Sholder Mount_v3 (Autodesk Fusion 360 design; units mm, degrees)
Autodesk Fusion 360 part; units mm, degrees
sketch "Sketch1" plane through (0, 0, 0) normal (0, 0, 1) x (1, 0, 0)
  circle A0 centre (0, 0) radius 65.25
  circle A1 centre (0, 0) radius 74.419 construction
  circle A2 centre (0, 74.419) radius 1.5
  circle A3 centre (-64.4487, -37.2095) radius 1.5
  circle A4 centre (64.4487, -37.2095) radius 1.5
  circle A5 centre (0, 0) radius 80
  line L0 (-80, 0) -> (80, 0) construction
  line L1 (-80, 0) -> (-80, -85)
  line L2 (80, -85) -> (80, 0)
  line L3 (-80, -95) -> (-100, -95) construction
  line L4 (-100, -95) -> (-90, -95)
  line L5 (100, -95) -> (100, -105)
  line L6 (100, -105) -> (-100, -105)
  line L7 (-100, -105) -> (-100, -95)
  arc A6 (-90, -95) -> (-80, -85) centre (-90, -85) ccw
  line L8 (90, -95) -> (100, -95)
  arc A7 (80, -85) -> (90, -95) centre (90, -85) ccw
  line L9 (-100, -100) -> (-30, -100) construction
  line L10 (-100, -100) -> (40, -100) construction
  circle A8 centre (-30, -100) radius 1.5
  circle A9 centre (40, -100) radius 1.5
  dimension "d1" = 130.5
  dimension "d4" = 148.838
  dimension "d5" = 3
  dimension "d7" = 360
  dimension "d8" = 160
  dimension "d10" = 200
  dimension "d11" = 10
  dimension "d12" = 10
  dimension "d13" = 10
  dimension "d22" = 105
  dimension "d24" = 70
  dimension "d25" = 140
  dimension "d26" = 3
  dimension "d27" = 3
  constraint coincident A0.centre A1.centre
  constraint concentric A0 A1
  constraint coincident A1 A2.centre
  constraint concentric A1 A5
  constraint coincident A5 L0.start
  constraint coincident A5 L0.end
  constraint horizontal L0
  constraint tangent A5 L1
  constraint perpendicular L0 L1
  constraint tangent A5 L2
  constraint perpendicular L1 L3
  constraint horizontal L4
  constraint vertical L5
  constraint horizontal L6
  constraint vertical L7
  constraint coincident L3.start L1
  constraint coincident L5.start L4
  constraint tangent L1 A6
  constraint tangent L4 A6
  constraint perpendicular L5 L8
  constraint tangent L8 A7
  constraint tangent L2 A7
  constraint midpoint L7 L9.start
  constraint perpendicular L7 L9
  constraint perpendicular L7 L10
  constraint coincident L9.end A8.centre
  constraint coincident L10.end A9.centre
  measures "d1" diameter of A0
  measures "d4" diameter of A1
  measures "d5" diameter of A2
  measures "d8" diameter of A5
  measures "d10" distance of L3.end L5.start
  measures "d11" distance of L3.end L6.end
  measures "d12" radius of A6 L3.start
  measures "d13" radius of A7
  measures "d22" distance of A0.centre L6
  measures "d24" distance of L9.start L9.end
  measures "d25" distance of L9.start L10.end
  measures "d26" diameter of A8
  measures "d27" diameter of A9
extrude "Extrude1" add sketch "Sketch1" along normal blind 10 contours A5 | A5 L1 L2 L4 L5 L6 L7 A6 L8 A7 | A8 | A9
hole "Hole1" at (-95, -95, 5) direction (0, -1, 0) diameter 3 depth 10 tip angle 118
hole "Hole2" at (95.1862, -95, 5.0204) direction (0, -1, 0) diameter 3 depth 10 tip angle 118
equation "d1 = GearboxDia + Tollerance"
equation "GearboxDia = 130 mm"
equation "Tollerance = 0.5 mm"
equation "d4 = ( 74.419 * 2 ) * 1 mm"
equation "d8 = GearboxDia + 30 mm"
equation "d10 = d8 + 40 mm"
equation "d22 = AxleHieght"
equation "AxleHieght = 105 mm"
equation "d24 = ( 210 / 3 ) * 1 mm"
equation "d25 = ( 210 / 3 * 2 ) * 1 mm"
